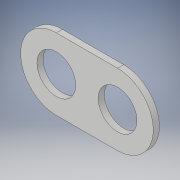
# Autodesk Inventor part: Inverter Housing Half 2
Saved by Autodesk Inventor 2019.4 (Build 234330000, 330)
## iProperties
Created: 2020-02-16
Part Number: Inverter Housing Half 2
Material: Generic
Document SubType Name: Modeling
Designer: admin
Density: 1 g/cm^3
Appearance: Default
Author: admin
Autodesk Inventor part; units mm, degrees
ref_plane "YZ Plane" through (0, 0, 0) normal (1, 0, 0) x (0, 1, 0)
ref_plane "XZ Plane" through (0, 0, 0) normal (0, 1, 0) x (-1, 0, 0)
ref_plane "XY Plane" through (0, 0, 0) normal (0, 0, 1) x (1, 0, 0)
sketch "Sketch1" plane through (0, 0, 0) normal (0, 0, 1) x (1, 0, 0)
  circle A0 centre (-15, 0) radius 9.5
  circle A1 centre (15, 0) radius 9.5
  line L0 (15, 0) -> (-15, 0) construction
  line L1 (-15, 0) -> (15, 0) construction
  line L2 (-15, -17.5) -> (15, -17.5)
  line L3 (15, 17.5) -> (-15, 17.5)
  arc A2 (-15, 17.5) -> (-15, -17.5) centre (-15, 0) ccw
  arc A3 (15, -17.5) -> (15, 17.5) centre (15, 0) ccw
  point P0 (0, 0)
  point P1 (0, 0)
  point P2 (0, 0)
  dimension "d0" = 19
  dimension "d1" = 19
  dimension "d2" = 30
  dimension "d3" = 35
  constraints: 10 end point, 4 centre point, 4 point on circle, 4 tangent, 2 equal length, 2 midpoint, 1 coincident, 1 horizontal
  measures "d0" diameter of A0
  measures "d1" diameter of A1
  measures "d2" distance of L0.end L0.start
  measures "d3" diameter of A3
extrude "Extrusion1" add sketch "Sketch1" along normal blind 3
body "Solid1"
